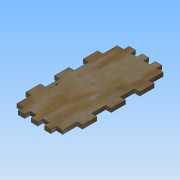
# Autodesk Inventor part: Base
Saved by Autodesk Inventor 2015 (Build 190159000, 159)
## iProperties
Created: 2014-11-11
Part Number: Base
Material: Generic
Document SubType Name: Modeling
Designer: 0
Density: 1 g/cm^3
Appearance: Plywood - Weathered
Mass: 92.3739 g
Surface Area: 335.328 cm^2
Volume: 92.3739 cm^3
BaseWidth: 6.560 in
BaseLength: 3.000 in
Thickness: 0.250 in
WallConSpace: 0.937 in
WallConA: 0.350 in
WallConB: 0.937 in
PerpSpace: 0.429 in
PerpB: 0.429 in
PerpA: 0.350 in
Author: 0
Autodesk Inventor part; units mm, degrees
ref_plane "YZ Plane" through (0, 0, 0) normal (1, 0, 0) x (0, 1, 0)
ref_plane "XZ Plane" through (0, 0, 0) normal (0, 1, 0) x (-1, 0, 0)
ref_plane "XY Plane" through (0, 0, 0) normal (0, 0, 1) x (1, 0, 0)
sketch "Sketch1" plane through (0, 0, 0) normal (0, 1, 0) x (-1, 0, 0)
  point P0 (0, 0)
sketch "Sketch2" plane through (0, 0, 0) normal (0, 1, 0) x (-1, 0, 0)
  line L0 (0, 0) -> (76.2, 0)
  line L1 (76.2, 0) -> (76.2, -166.624)
  line L2 (76.2, -166.624) -> (0, -166.624)
  line L3 (0, -166.624) -> (0, 0)
  dimension "BaseLength" = 76.2
  dimension "BaseWidth" = 166.624
  constraints: 8 end point, 2 parallel, 1 horizontal, 1 perpendicular
  measures "BaseLength" distance of L1.end L2.end
  measures "BaseWidth" distance of L0.end L1.end
extrude "Base Extrusion" add sketch "Sketch2" along normal blind 6.35
sketch "Sketch3" plane through (0, 0, 0) normal (0, 1, 0) x (-1, 0, 0)
  line L0 (76.2, 0) -> (0, 0) projected
  line L1 (0, 0) -> (0, -166.624) projected
  line L2 (0, -166.624) -> (76.2, -166.624) projected
  line L3 (76.2, -166.624) -> (76.2, 0) projected
  line L4 (10.8857, 0) -> (21.7714, 0)
  line L5 (21.7714, 0) -> (21.7714, 8.89)
  line L6 (21.7714, 8.89) -> (10.8857, 8.89)
  line L7 (10.8857, 8.89) -> (10.8857, 0)
  line L8 (32.6571, 0) -> (43.5429, 0)
  line L9 (43.5429, 0) -> (43.5429, 8.89)
  line L10 (43.5429, 8.89) -> (32.6571, 8.89)
  line L11 (32.6571, 8.89) -> (32.6571, 0)
  line L12 (54.4286, 0) -> (65.3143, 0)
  line L13 (65.3143, 0) -> (65.3143, 8.89)
  line L14 (65.3143, 8.89) -> (54.4286, 8.89)
  line L15 (54.4286, 8.89) -> (54.4286, 0)
  line L16 (76.2, -83.312) -> (0, -83.312) construction
  line L17 (76.2, -166.624) -> (0, -166.624)
  line L18 (10.8857, -166.624) -> (21.7714, -166.624)
  line L19 (21.7714, -166.624) -> (21.7714, -175.514)
  line L20 (21.7714, -175.514) -> (10.8857, -175.514)
  line L21 (10.8857, -175.514) -> (10.8857, -166.624)
  line L22 (43.5429, -166.624) -> (43.5429, -175.514)
  line L23 (43.5429, -175.514) -> (32.6571, -175.514)
  line L24 (32.6571, -175.514) -> (32.6571, -166.624)
  line L25 (32.6571, -166.624) -> (43.5429, -166.624)
  line L26 (65.3143, -166.624) -> (65.3143, -175.514)
  line L27 (65.3143, -175.514) -> (54.4286, -175.514)
  line L28 (54.4286, -175.514) -> (54.4286, -166.624)
  line L29 (54.4286, -166.624) -> (65.3143, -166.624)
  line L30 (38.1, 0) -> (38.1, -166.624) construction
  line L31 (0, -23.8034) -> (-8.89, -23.8034)
  line L32 (-8.89, -23.8034) -> (-8.89, -47.6069)
  line L33 (-8.89, -47.6069) -> (0, -47.6069)
  line L34 (0, -47.6069) -> (0, -23.8034)
  line L35 (0, -71.4103) -> (-8.89, -71.4103)
  line L36 (-8.89, -71.4103) -> (-8.89, -95.2137)
  line L37 (-8.89, -95.2137) -> (0, -95.2137)
  line L38 (0, -95.2137) -> (0, -71.4103)
  line L39 (0, -119.0171) -> (-8.89, -119.0171)
  line L40 (-8.89, -119.0171) -> (-8.89, -142.8206)
  line L41 (-8.89, -142.8206) -> (0, -142.8206)
  line L42 (0, -142.8206) -> (0, -119.0171)
  line L43 (76.2, 0) -> (76.2, -166.624)
  line L44 (76.2, -23.8034) -> (85.09, -23.8034)
  line L45 (85.09, -23.8034) -> (85.09, -47.6069)
  line L46 (85.09, -47.6069) -> (76.2, -47.6069)
  line L47 (76.2, -47.6069) -> (76.2, -23.8034)
  line L48 (76.2, -71.4103) -> (85.09, -71.4103)
  line L49 (85.09, -71.4103) -> (85.09, -95.2137)
  line L50 (85.09, -95.2137) -> (76.2, -95.2137)
  line L51 (76.2, -95.2137) -> (76.2, -71.4103)
  line L52 (76.2, -119.0171) -> (85.09, -119.0171)
  line L53 (85.09, -119.0171) -> (85.09, -142.8206)
  line L54 (85.09, -142.8206) -> (76.2, -142.8206)
  line L55 (76.2, -142.8206) -> (76.2, -119.0171)
  dimension "d4" = 10.8857
  dimension "d5" = 8.89
  dimension "PerpSpace" = 10.8857
  dimension "d7" = 10.8857
  dimension "d8" = 8.89
  dimension "PerpB" = 10.8857
  dimension "PerpA" = 8.89
  dimension "d11" = 10.8857
  dimension "d13" = 10.8857
  dimension "d14" = 76.2
  dimension "WallConSpace" = 23.8034
  dimension "d16" = 166.624
  dimension "WallConA" = 8.89
  dimension "WallConB" = 23.8034
  dimension "d19" = 8.89
  dimension "d20" = 23.8034
  dimension "d21" = 8.89
  dimension "d22" = 23.8034
  dimension "d23" = 23.8034
  dimension "d24" = 23.8034
  constraints: 104 end point, 24 symmetric about line, 12 parallel, 6 collinear, 6 horizontal, 6 perpendicular, 4 midpoint
  measures "d4" distance of L6.end L5.end
  measures "d5" distance of L5.end L4.end
  measures "PerpSpace" distance between parallel lines of L1 L7
  measures "d7" distance of L10.end L9.end
  measures "d8" distance of L9.end L9.start
  measures "PerpB" distance of L14.end L13.end
  measures "PerpA" distance of L13.end L13.start
  measures "d11" distance between parallel lines of L5 L11
  measures "d13" distance between parallel lines of L9 L15
  measures "d14" distance of L0.start L0.end
  measures "WallConSpace" distance between parallel lines of L0 L31
  measures "d16" distance of L0.end L1.end
  measures "WallConA" distance of L32.end L33.end
  measures "WallConB" distance of L31.end L32.end
  measures "d19" distance of L35.start L35.end
  measures "d20" distance of L35.end L36.end
  measures "d21" distance of L39.start L39.end
  measures "d22" distance of L39.end L40.end
  measures "d23" distance between parallel lines of L33 L35
  measures "d24" distance between parallel lines of L37 L39
extrude "Connections" add sketch "Sketch3" along normal blind 6.35 contours L0 L15 L14 L13 | L44 L45 L46 L3 | L0 L11 L10 L9 | L48 L49 L50 L3 | L0 L7 L6 L5 | L52 L53 L54 L3 | L1 L33 L32 L31 | L26 L27 L28 L2 | L1 L37 L36 L35 | L22 L23 L24 L2 | L1 L41 L40 L39 | L19 L20 L21 L2
sketch "Notes" plane through (0, 6.35, 0) normal (0, 1, 0) x (1, 0, 0)
  line L0 (-72.1433, 48.3233) -> (-72.1433, 70.3861) construction
  line L1 (-72.1433, 70.3861) -> (-23.5271, 70.3861) construction
  line L2 (-23.5271, 70.3861) -> (-23.5271, 48.3233) construction
  line L3 (-23.5271, 48.3233) -> (-72.1433, 48.3233) construction
  point P0 (0, 0)
  constraints: 2 other
equation "\"d4\" = 0.142857 * d14"
equation "\"PerpSpace\" = -0.75 * d4 + 0.25 * d14"
equation "\"d7\" = d4"
equation "\"d8\" = d5"
equation "\"PerpB\" = d4"
equation "\"PerpA\" = d5"
equation "\"d11\" = PerpSpace"
equation "\"d13\" = PerpSpace"
equation "\"WallConSpace\" = -0.75 * WallConB + 0.25 * d16"
equation "\"WallConB\" = 0.142857 * d16"
equation "\"d19\" = WallConA"
equation "\"d20\" = WallConB"
equation "\"d21\" = WallConA"
equation "\"d22\" = WallConB"
equation "\"d23\" = WallConSpace"
equation "\"d24\" = WallConSpace"
body "Solid1"
